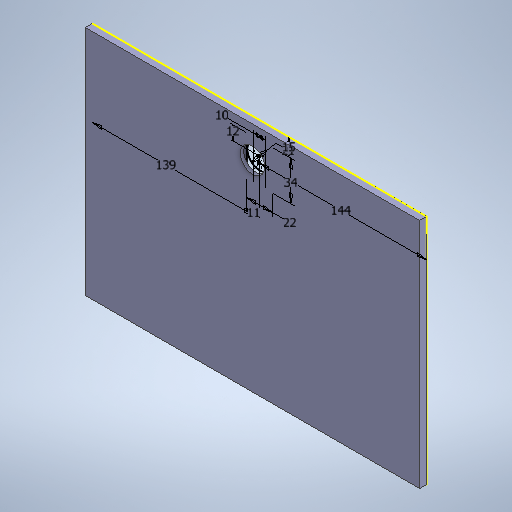
# Autodesk Inventor part: RightWall
Saved by Autodesk Inventor 2026.2 (Build 302298010, 298A)
## iProperties
Created: 2026-03-19
Part Number: RightWall
Material: Ogólny
Document SubType Name: Modeling
Designer: Patryk
Density: 1 g/cm^3
Appearance: Domyślna
Author: Patryk
Autodesk Inventor part; units mm, degrees
ref_plane "YZ Plane" through (0, 0, 0) normal (1, 0, 0) x (0, 1, 0)
ref_plane "XZ Plane" through (0, 0, 0) normal (0, 1, 0) x (-1, 0, 0)
ref_plane "XY Plane" through (0, 0, 0) normal (0, 0, 1) x (1, 0, 0)
sketch "Szkic1" plane through (0, 0, 0) normal (0, 0, 1) x (1, 0, 0)
  line L0 (144, 100) -> (-144, 100)
  line L1 (-144, 100) -> (-144, -100)
  line L2 (-144, -100) -> (144, -100)
  line L3 (144, -100) -> (144, 100)
  line L4 (144, 100) -> (-144, -100) construction
  line L5 (-144, 100) -> (144, -100) construction
  point P0 (0, 0)
  dimension "d0" = 288
  dimension "d1" = 200
  constraints: 12 end point, 2 midpoint, 2 parallel, 1 horizontal, 1 perpendicular
  measures "d0" distance of L2.end L1.end
  measures "d1" distance of L1.end L0.end
extrude "Wyciągnięcie proste1" add sketch "Szkic1" along normal mid plane 6
sketch "Szkic2" plane through (0, 0, -3) normal (0, 0, -1) x (-1, 0, 0)
  line L0 (11, 51) -> (-11, 51)
  line L1 (-11, 51) -> (-11, 85)
  line L2 (-11, 85) -> (11, 85)
  line L3 (11, 85) -> (11, 51)
  line L4 (11, 51) -> (-11, 85) construction
  line L5 (-11, 51) -> (11, 85) construction
  line L6 (144, 100) -> (-144, 100) projected
  line L7 (-144, 100) -> (-144, -100) projected
  circle A0 centre (0, 73) radius 10.5
  line L8 (-144, -100) -> (144, -100) projected
  line L9 (144, -100) -> (144, 100) projected
  line L10 (-5, 51) -> (-5, -100)
  line L11 (5, 51) -> (5, -100)
  point P0 (0, 0)
  point P1 (0, 68)
  dimension "d4" = 34
  dimension "d5" = 22
  dimension "d6" = 15
  dimension "d8" = 21
  dimension "d9" = 12
  dimension "d10" = 11
  dimension "d15" = 10
  dimension "d16" = 139
  dimension "d19" = 144
  constraints: 16 end point, 4 point on line, 2 midpoint, 2 parallel, 2 perpendicular, 1 centre point, 1 horizontal, 1 vertical
  measures "d4" distance of L0.end L1.end
  measures "d5" distance of L0.start L0.end
  measures "d6" distance between parallel lines of L6 L2
  measures "d8" diameter of A0
  measures "d9" distance from line of L2 A0.centre
  measures "d10" distance from line of L3 A0.centre
  measures "d15" distance between parallel lines of L11 L10
  measures "d16" distance between parallel lines of L9 L11
  measures "d19" distance from line of A0.centre L7
extrude "Wyciągnięcie proste2" cut sketch "Szkic2" against normal through all contours A0
extrude "Wyciągnięcie proste3" cut sketch "Szkic2" against normal blind 3 contours L0 L1 L2 L3
extrude "Wyciągnięcie proste5" cut sketch "Szkic2" against normal blind 3 contours L11 L8 L10 L0
